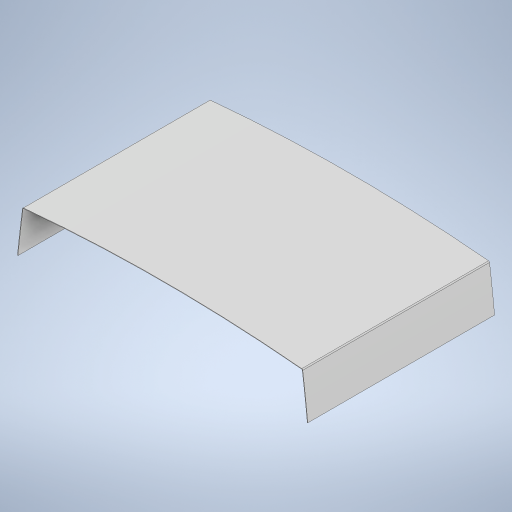
# Autodesk Inventor part: МОО 010 лист спина 1
Saved by Autodesk Inventor 2024.2 (Build 282272000, 272)
## iProperties
Created: 2024-04-18
Part Number: МОО 010 лист спина 1
Material: Stainless Steel AISI 304
Document SubType Name: Sheet Metal
Designer: admin
Density: 8 g/cm^3
Sheet Metal Rule: Default_mm
Sheet Metal Width: 0,000 mm
Sheet Metal Length: 0,000 mm
Sheet Metal Area: 0,000 mm^2
Appearance: Default
Mass: 48037.2 g
Surface Area: 40211.1 cm^2
Volume: 6004.65 cm^3
Stock Number: МОО 010 лист спина 1
Author: admin
Autodesk Inventor part; units mm, degrees
note: some values were not read from the file. Chosen so that the rebuilt part matches the saved one: flange form of "Plate1".
ref_plane "YZ Plane" through (0, 0, 0) normal (1, 0, 0) x (0, 1, 0)
ref_plane "XZ Plane" through (0, 0, 0) normal (0, 1, 0) x (-1, 0, 0)
ref_plane "XY Plane" through (0, 0, 0) normal (0, 0, 1) x (1, 0, 0)
sketch "Sketch1" plane through (0, 0, 0) normal (0, 0, 1) x (1, 0, 0)
  line L0 (-750, 0) -> (750, 0) construction
  line L1 (750, 0) -> (750, -2100) construction
  line L2 (750, -2100) -> (110, -2700) construction
  line L3 (108.9077, -2700) -> (-108.9077, -2700) construction
  line L4 (-110, -2700) -> (-750, -2100) construction
  line L5 (-750, -2100) -> (-750, 0) construction
  arc A0 (745.2369, 0.4471) -> (-745.2369, 0.4471) centre (0, -7964.7662) ccw
  arc A1 (-750.6265, -4.7429) -> (-776.2932, -222.5) centre (7180.7944, -1050) ccw
  arc A2 (-777.5832, -235) -> (-778.8534, -247.5) centre (7180.7944, -1050) ccw construction
  arc A3 (750.1285, -2099.0286) -> (778.8534, -247.5) centre (-7180.7944, -1050) ccw construction
  arc A4 (777.5832, -235) -> (776.2932, -222.5) centre (-7180.7944, -1050) ccw
  line L6 (-777.5832, -235) -> (777.5832, -235) construction
  arc A5 (-749.3229, -2100.7083) -> (-677.5699, -2174.8011) centre (5033.2984, 3427.5183) ccw construction
  line L7 (-750, -2100) -> (750, -2100) construction
  line L8 (-547.1729, -2035.7109) -> (-801.0834, -2306.5488) construction
  arc A6 (-677.5699, -2174.8011) -> (-110.8367, -2699.2976) centre (5033.2984, 3427.5183) ccw construction
  arc A7 (-745.2369, 0.4471) -> (-750.6265, -4.7429) centre (-744.6779, -5.5268) ccw
  arc A8 (750.6265, -4.7429) -> (745.2369, 0.4471) centre (744.6779, -5.5268) ccw
  arc A9 (-750.1285, -2099.0286) -> (-749.3229, -2100.7083) centre (-747.1545, -2098.6352) ccw construction
  arc A10 (110.8367, -2699.2976) -> (677.5699, -2174.8011) centre (-5033.2984, 3427.5183) ccw construction
  line L9 (553.8195, -2042.8006) -> (794.4368, -2299.4591) construction
  arc A11 (677.5699, -2174.8011) -> (749.3229, -2100.7083) centre (-5033.2984, 3427.5183) ccw construction
  arc A12 (749.3229, -2100.7083) -> (750.1285, -2099.0286) centre (747.1545, -2098.6352) ccw construction
  arc A13 (-110.8367, -2699.2976) -> (-108.9077, -2700) centre (-108.9077, -2697) ccw construction
  arc A14 (108.9077, -2700) -> (110.8367, -2699.2976) centre (108.9077, -2697) ccw construction
  line L10 (-778.8534, -247.5) -> (778.8534, -247.5) construction
  line L11 (-776.2932, -222.5) -> (776.2932, -222.5) construction
  arc A15 (-776.2932, -222.5) -> (-777.5832, -235) centre (7180.7944, -1050) ccw
  arc A16 (-778.8534, -247.5) -> (-750.1285, -2099.0286) centre (7180.7944, -1050) ccw construction
  arc A17 (778.8534, -247.5) -> (777.5832, -235) centre (-7180.7944, -1050) ccw construction
  arc A18 (776.2932, -222.5) -> (750.6265, -4.7429) centre (-7180.7944, -1050) ccw
  point P0 (0, 0)
  point P1 (0, 0)
  point P2 (0, -2700)
  point P3 (-674.1281, -2171.1299)
  point P4 (674.1281, -2171.1299)
  dimension "d17" = 1500
  dimension "d18" = 2100
  dimension "d19" = 220
  dimension "d20" = 2700
  dimension "d21" = 8000
  dimension "d31" = 8000
  dimension "d33" = 8000
  dimension "d34" = 235
  dimension "d35" = 8000
  dimension "d36" = 104
  dimension "d37" = 6
  dimension "d40" = 3
  dimension "d41" = 8000
  dimension "d42" = 104
  dimension "d44" = 3
  dimension "d46" = 12.5
  dimension "d47" = 12.5
  measures "d17" distance of L0.end L0.start
  measures "d18" distance of L1.end L0.end
  measures "d19" distance of L2.end L4.start
  measures "d20" vertical distance of point (0, -2700) L0.start
  measures "d21" radius of A0
  measures "d31" radius of A1
  measures "d33" radius of A3
  measures "d34" distance between parallel lines of L0 L6
  measures "d35" radius of A5
  measures "d36" distance of L4.end point (-674.128, -2171.13)
  measures "d37" radius of A7
  measures "d40" radius of A9
  measures "d41" radius of A10
  measures "d42" distance of L1.end point (674.128, -2171.13)
  measures "d44" radius of A13
  measures "d46" distance between parallel lines of L10 L6
  measures "d47" distance between parallel lines of L11 L6
contour flange "Contour Flange1" sketch "Sketch1" thickness 3 bend radius 3 width 1000 along (0, 0, 1) mid plane no both sides no wall seen from (776.9407, -228.7497, 0) lies toward (-0.9947169, -0.1026563, 0) curves A4 A18 A8 A0 A7 A1 A15
bend "Bend1"
corner "Corner1"
equation "\"d17\" = Бак_ширина_общая"
equation "\"d18\" = Бак_высота_до_конуса"
equation "\"d19\" = Бак_брюхо_ширина_полки"
equation "\"d20\" = Бак_высота_общая"
equation "\"d21\" = Бак_радиус_стенок_общий"
equation "\"d31\" = Бак_радиус_стенок_общий"
equation "\"d33\" = Бак_радиус_стенок_общий"
equation "\"d34\" = Бак_спина_длина_фланцев"
equation "\"d35\" = Бак_радиус_стенок_общий"
equation "\"d36\" = Бак_борт_длина_фланца"
equation "\"d37\" = Thickness + BendRadius"
equation "\"d40\" = Thickness"
equation "\"d41\" = Бак_радиус_стенок_общий"
equation "\"d42\" = d36"
equation "\"d46\" = Бак_нахлест_фланца"
equation "\"d47\" = Бак_нахлест_фланца"
equation "\"d3\" = Thickness"
equation "\"d4\" = BendReliefWidth"
equation "\"d5\" = BendReliefDepth"
equation "\"d6\" = MinimumRemnant"
equation "\"d7\" = TransitionRadius"
equation "\"d9\" = BendRadius"
equation "\"d11\" = CornerReliefSize"
equation "\"d12\" = GapSize"
equation "\"d13\" = JacobiRadiusSize"
equation "\"BendRadius\" = Thickness"
equation "\"BendReliefWidth\" = Thickness"
equation "\"BendReliefDepth\" = 0.5 * Thickness"
equation "\"CornerReliefSize\" = 4 * Thickness"
equation "\"MinimumRemnant\" = 2 * Thickness"
equation "\"TransitionRadius\" = BendRadius"
equation "\"JacobiRadiusSize\" = BendRadius"
equation "\"GapSize\" = Thickness"
equation "\"Бак_ширина_общая\" = 1500"
equation "\"Бак_высота_до_конуса\" = 2100"
equation "\"Бак_брюхо_ширина_полки\" = 220"
equation "\"Бак_радиус_стенок_общий\" = 8000"
equation "\"Бак_спина_длина_фланцев\" = 235"
equation "\"Thickness\" = 3"
equation "\"Бак_нахлест_фланца\" = 12.5"
equation "\"Бак_высота_общая\" = 2700"
equation "\"Бак_борт_длина_фланца\" = 104"
body "Solid1"
